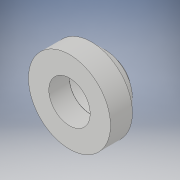
# Autodesk Inventor part: motor_and_magnet_holder
Saved by Autodesk Inventor 2019.4 (Build 234330000, 330)
## iProperties
Created: 2019-06-20
Part Number: motor_and_magnet_holder
Material: Generic
Document SubType Name: Modeling
Designer: cdi
Density: 1 g/cm^3
Appearance: Default
Author: cdi
Autodesk Inventor part; units mm, degrees
ref_plane "YZ Plane" through (0, 0, 0) normal (1, 0, 0) x (0, 1, 0)
ref_plane "XZ Plane" through (0, 0, 0) normal (0, 1, 0) x (-1, 0, 0)
ref_plane "XY Plane" through (0, 0, 0) normal (0, 0, 1) x (1, 0, 0)
sketch "Sketch1" plane through (0, 0, 0) normal (0, 0, 1) x (1, 0, 0)
  circle A0 centre (0, 0) radius 6
  dimension "d0" = 12
  constraints: 1 centre point, 1 coincident
  measures "d0" diameter of A0
extrude "Extrusion1" add sketch "Sketch1" along normal blind 3.5
sketch "Sketch2" plane through (0, 0, 3.5) normal (0, 0, 1) x (1, 0, 0)
  circle A0 centre (0, 0) radius 1.55
  dimension "d3" = 3.1
  constraints: 1 centre point, 1 coincident
  measures "d3" diameter of A0
extrude "Extrusion2" cut sketch "Sketch2" against normal through all
sketch "Sketch3" plane through (0, 0, 0) normal (0, 0, -1) x (-1, 0, 0)
  circle A0 centre (0, 0) radius 2.96
  circle A1 centre (0, 0) radius 7.5
  dimension "d6" = 5.92
  dimension "d16" = 15
  constraints: 2 centre point, 2 coincident
  measures "d6" diameter of A0
  measures "d16" diameter of A1
extrude "Extrusion3" cut sketch "Sketch3" against normal blind 0.8
sketch "Sketch4" plane through (0, 0, 3.5) normal (0, 0, 1) x (1, 0, 0)
  circle A0 centre (0, 0) radius 2.5
  dimension "d9" = 5
  constraints: 1 centre point, 1 coincident
  measures "d9" diameter of A0
extrude "Extrusion4" cut sketch "Sketch4" against normal blind 1.5
sketch "Sketch5" plane through (0, 0, 3.5) normal (0, 0, 1) x (1, 0, 0)
  circle A0 centre (0, 0) radius 6
  circle A1 centre (0, 0) radius 2.5 projected
  circle A2 centre (0, 0) radius 3.025
  circle A3 centre (0, 0) radius 6 projected
  dimension "d12" = 6.05
  dimension "d15" = 0
  constraints: 2 centre point, 2 coincident
  measures "d12" diameter of A2
  measures "d15" radial gap between concentric circles of A3 A0
extrude "Extrusion5" add sketch "Sketch5" along normal blind 2.5 contours A0
chamfer "Chamfer1" distance 2 angle 45 1 edges at (-6, 0, 0.8)
sketch "Sketch6" plane through (0, 0, 3.5) normal (0, 0, 1) x (1, 0, 0)
  circle A0 centre (0, 0) radius 3.025 projected
  circle A1 centre (0, 0) radius 2.5 projected
extrude "Extrusion6" cut sketch "Sketch6" against normal up to surface (1.5 mm away)
sketch "Sketch7" plane through (0, 0, 2) normal (0, 0, 1) x (1, 0, 0)
  circle A0 centre (0, 0) radius 3.025 projected
  circle A1 centre (0, 0) radius 1.55 projected
extrude "Extrusion7" add sketch "Sketch7" along normal blind 1
sketch "Sketch8" plane through (0, 0, 3) normal (0, 0, 1) x (1, 0, 0)
  point P0 (0, 0)
hole "Hole1" at (0, 0, 3) direction (0, 0, -1) diameter 3.2 end through all countersink diameter 6 countersink angle 90
body "Solid1"
